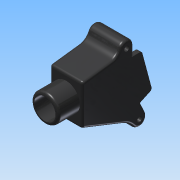
# Autodesk Inventor part: Rear Axle Housing
Saved by Autodesk Inventor 2014 (Build 180170000, 170)
## iProperties
Created: 2014-01-04
Part Number: Rear Axle Housing
Material: ABS Plastic
Document SubType Name: Modeling
Designer: davidgitz
Density: 1.06 g/cm^3
Appearance: Dark Gray
Author: davidgitz
Autodesk Inventor part; units mm, degrees
ref_plane "YZ Plane" through (0, 0, 0) normal (1, 0, 0) x (0, 1, 0)
ref_plane "XZ Plane" through (0, 0, 0) normal (0, 1, 0) x (-1, 0, 0)
ref_plane "XY Plane" through (0, 0, 0) normal (0, 0, 1) x (1, 0, 0)
sketch "Sketch1" plane through (0, 0, 0) normal (1, 0, 0) x (0, 1, 0)
  circle A0 centre (41.2183, 7.8588) radius 1.4732
  circle A1 centre (0, 0) radius 1.4732
  arc A2 (41.2183, 3.5408) -> (43.1083, 11.7412) centre (41.2183, 7.8588) ccw
  arc A3 (-2.7625, 3.3187) -> (1.8095, -3.9206) centre (0, 0) ccw
  line L0 (12.0367, -7.5928) -> (8.8435, -0.6741)
  line L1 (8.8435, -0.6741) -> (1.8095, -3.9206)
  line L2 (12.0367, -7.5928) -> (35.345, -1.3496)
  line L3 (-6.175, 3.0752) -> (5.5506, -22.3305) construction
  line L4 (12.0367, -7.5928) -> (0, 0) construction
  line L5 (0, 0) -> (41.2183, 7.8588) construction
  line L6 (12.0367, -7.5928) -> (41.2183, 7.8588) construction
  line L7 (41.2183, 7.8588) -> (35.345, -1.3496) construction
  line L8 (41.2183, 3.5408) -> (35.345, 3.5408)
  line L9 (35.345, -1.3496) -> (35.345, 3.5408)
  line L10 (12.2353, 34.8247) -> (36.5685, 34.8247)
  line L11 (35.345, -1.3496) -> (36.5685, 34.8247) construction
  line L12 (12.2353, 34.8247) -> (12.0367, -7.5928) construction
  line L13 (12.2353, 34.8247) -> (35.345, -1.3496) construction
  line L14 (-2.7625, 3.3187) -> (-1.4733, 4.3919)
  line L15 (2.2114, 9.4815) -> (12.2353, 34.8247)
  arc A4 (-1.4733, 4.3919) -> (2.2114, 9.4815) centre (-9.5984, 14.1526) ccw
  line L16 (36.5685, 34.8247) -> (38.8252, 17.0234)
  line L17 (42.3454, 12.1126) -> (43.1083, 11.7412)
  arc A5 (38.8252, 17.0234) -> (42.3454, 12.1126) centre (45.1248, 17.822) ccw
  dimension "d0" = 2.9464
  dimension "d1" = 8.636
  dimension "d2" = 24.13
  dimension "d3" = 7.62
  dimension "d4" = 12.065
  dimension "d5" = 14.2314
  dimension "d6" = 41.9608
  dimension "d7" = 33.02
  dimension "d8" = 10.922
  dimension "d9" = 24.3332
  dimension "d10" = 36.195
  dimension "d11" = 42.418
  dimension "d12" = 42.926
  dimension "d17" = 15
  dimension "d20" = 12.7
  dimension "d21" = 6.35
  constraints: 36 end point, 9 tangent, 8 point on circle, 6 centre point, 4 perpendicular, 3 coincident, 2 equal radius, 1 horizontal
  measures "d0" diameter of A0
  measures "d1" diameter of A2
  measures "d2" distance of L0.start L2.end
  measures "d3" distance of L0.start L0.end
  measures "d4" distance between parallel lines of L3 L0
  measures "d5" distance of L0.start L4.end
  measures "d6" distance of L4.end L5.end
  measures "d7" distance of L0.start L5.end
  measures "d8" distance of L5.end L2.end
  measures "d9" distance of L10.start L10.end
  measures "d10" distance of L2.end L10.end
  measures "d11" distance of L10.start L0.start
  measures "d12" distance of L10.start L2.end
  measures "d17" angle of L1 L14
  measures "d20" radius of A4
  measures "d21" radius of A5
extrude "Extrusion1" add sketch "Sketch1" along normal mid plane 20.066
sketch "Sketch2" plane through (-10.033, 12.2353, 34.8247) normal (0, 0, 1) x (1, 0, 0)
  line L0 (0, 24.3332) -> (20.066, 0) construction
  circle A0 centre (10.033, 12.1666) radius 8.4201
  circle A1 centre (10.033, 12.1666) radius 6.477
  point P0 (10.033, -12.2353)
  dimension "d22" = 16.8402
  dimension "d23" = 12.954
  constraints: 2 centre point, 2 end point, 1 coincident, 1 midpoint
  measures "d22" diameter of A0
  measures "d23" diameter of A1
extrude "Extrusion2" add sketch "Sketch2" along normal blind 12.954
sketch "Sketch4" plane through (0, 0, 0) normal (1, 0, 0) x (0, 1, 0)
  line L0 (36.5685, 34.8247) -> (38.8252, 17.0234) projected
  circle A0 centre (0, 0) radius 1.4732 projected
  circle A1 centre (41.2183, 7.8588) radius 1.4732 projected
  line L1 (12.0367, -7.5928) -> (8.8435, -0.6741) projected
  line L2 (8.8435, -0.6741) -> (1.8095, -3.9206) projected
  arc A2 (-2.7625, 3.3187) -> (1.8095, -3.9206) centre (0, 0) ccw projected
  line L3 (-2.7625, 3.3187) -> (-1.4733, 4.3919) projected
  arc A3 (-1.4733, 4.3919) -> (2.2114, 9.4815) centre (-9.5984, 14.1526) ccw projected
  line L4 (2.2114, 9.4815) -> (12.2353, 34.8247) projected
  line L5 (12.2353, 34.8247) -> (36.5685, 34.8247) projected
  line L6 (36.5685, 34.8247) -> (38.8252, 17.0234) projected
  arc A4 (38.8252, 17.0234) -> (42.3454, 12.1126) centre (45.1248, 17.822) ccw projected
  line L7 (42.3454, 12.1126) -> (43.1083, 11.7412) projected
  arc A5 (41.2183, 3.5408) -> (43.1083, 11.7412) centre (41.2183, 7.8588) ccw projected
  line L8 (41.2183, 3.5408) -> (35.345, 3.5408) projected
  line L9 (35.345, 3.5408) -> (35.345, -1.3496) projected
  line L10 (35.345, -1.3496) -> (12.0367, -7.5928) projected
  line L11 (37.22, 9.4895) -> (34.3301, 32.2847)
  line L12 (34.3301, 32.2847) -> (13.9621, 32.2847)
  line L13 (13.9621, 32.2847) -> (2.5662, 3.4727)
  arc A6 (0.5201, -1.7002) -> (0.7451, -1.6144) centre (0, 0) ccw
  arc A7 (37.22, 9.4895) -> (44.3293, 4.8643) centre (41.2183, 7.8588) ccw
  arc A8 (0.5042, -4.2885) -> (2.5662, 3.4727) centre (0, 0) ccw
  line L14 (46.3383, 2.4508) -> (-0.4795, -17.454)
  line L15 (-0.4795, -17.454) -> (0.5042, -4.2885)
  line L16 (46.3383, 2.4508) -> (44.3293, 4.8643)
  dimension "d26" = 2.54
  constraints: 14 end point, 8 point on circle, 3 centre point, 2 coincident, 2 concentric, 1 point on line
  measures "d26" distance between parallel lines of L0 L11
extrude "Extrusion3" cut sketch "Sketch4" along normal mid plane 14.732 contours L16 L14 L15 A2 L2 L1 L10 L9 L8 A5 | L8 L9 L10 L1 L2 A8 L13 L12 L11 A7
sketch "Sketch5" plane through (7.366, 34.3301, 32.2847) normal (0, 0, -1) x (-1, 0, 0)
  circle A0 centre (7.366, -9.9283) radius 6.477 projected
  circle A1 centre (7.366, -9.9283) radius 8.4201 projected
  point P0 (7.366, -34.3301)
extrude "Extrusion4" cut sketch "Sketch5" against normal up to next contours A0
fillet "Fillet1" radius 1.5875 29 edges at (10.033, 39.9638, 14.1225) (10.033, 42.7269, 11.9269) (10.033, 45.426, 6.889) (10.033, 38.2817, 3.5408) (10.033, 37.6969, 25.924) (0, 36.5685, 34.8247) (10.033, 24.4019, 34.8247) (10.033, 0.6888, 6.7052) (10.033, -2.1179, 3.8553) (10.033, -3.6508, -2.3057) (10.033, 5.3265, -2.2974) (10.033, 7.2233, 22.1531) (-10.033, 24.4019, 34.8247) (0, 12.2353, 34.8247) (-10.033, 0.6888, 6.7052) (-10.033, -2.1179, 3.8553) (-10.033, -3.6508, -2.3057) (-10.033, 5.3265, -2.2974) (-10.033, 7.2233, 22.1531) (-10.033, 39.9638, 14.1225) (-10.033, 42.7269, 11.9269) (-10.033, 45.426, 6.889) (-10.033, 38.2817, 3.5408) (-10.033, 37.6969, 25.924) (8.6995, 35.345, -1.3496) (-8.6995, 35.345, -1.3496) (8.6995, 12.0367, -7.5928) (-8.6995, 12.0367, -7.5928) (-8.4201, 24.4019, 47.7787)
body "Solid1"
